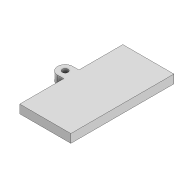
# Autodesk Inventor part: Ortak_bat_lid
Saved by Autodesk Inventor 2022 (Build 260153000, 153)
## iProperties
Created: 2023-02-07
Part Number: Ortak_bat_lid
Material: Generic
Document SubType Name: Modeling
Designer: MVeszpremi
Density: 1 g/cm^3
Appearance: Default
Author: MVeszpremi
Autodesk Inventor part; units mm, degrees
ref_plane "YZ Plane" through (0, 0, 0) normal (1, 0, 0) x (0, 1, 0)
ref_plane "XZ Plane" through (0, 0, 0) normal (0, 1, 0) x (-1, 0, 0)
ref_plane "XY Plane" through (0, 0, 0) normal (0, 0, 1) x (1, 0, 0)
sketch "Sketch1" plane through (0, 0, 0) normal (0, 1, 0) x (-1, 0, 0)
  line L0 (13.5, 27.25) -> (-13.5, 27.25)
  line L1 (-13.5, 27.25) -> (-13.5, -27.25)
  line L2 (-13.5, -27.25) -> (13.5, -27.25)
  line L3 (13.5, -27.25) -> (13.5, 27.25)
  line L4 (13.5, 27.25) -> (-13.5, -27.25) construction
  line L5 (-13.5, 27.25) -> (13.5, -27.25) construction
  circle A0 centre (16.75, 0) radius 1.5
  circle A1 centre (16.75, 0) radius 4
  line L6 (20.75, -4) -> (12.75, -4)
  line L7 (12.75, -4) -> (12.75, 4)
  line L8 (12.75, 4) -> (20.75, 4)
  line L9 (20.75, 4) -> (20.75, -4)
  line L10 (20.75, -4) -> (12.75, 4) construction
  line L11 (12.75, -4) -> (20.75, 4) construction
  point P0 (0, 0)
  point P1 (16.75, -4)
  point P2 (16.75, 4)
  point P3 (13.5, 4)
  point P4 (13.5, -4)
  dimension "d0" = 54.5
  dimension "d1" = 27
  dimension "d3" = 3
  dimension "d4" = 8
  dimension "d7" = 3.25
  constraints: 24 end point, 4 midpoint, 4 parallel, 2 centre point, 2 horizontal, 2 perpendicular, 1 coincident, 1 tangent
  measures "d0" distance of L2.end L0.start
  measures "d1" distance of L1.end L2.end
  measures "d3" diameter of A0
  measures "d4" diameter of A1
  measures "d7" distance from line of L3 A0.centre
extrude "Extrusion1" add sketch "Sketch1" along normal blind 4.5 contours L3 L8 L7 L6 L2 L1 L0 | L8 A1 L3 | L3 A1 L7 L8 | A1 L3 | L3 A1 | A1 L6 L3 | L3 L6 L7 A1
body "Solid1"
